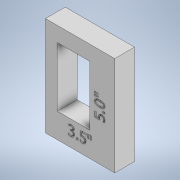
# Autodesk Inventor part: rectangular3_5x5_0-in-Template
Saved by Autodesk Inventor 2020.2 (Build 242310000, 310)
## iProperties
Created: 2020-01-27
Part Number: rectangular3_5x5_0-in-Template
Material: Generic
Document SubType Name: Modeling
Designer: robst
Density: 1 g/cm^3
Appearance: Default
Author: robst
Autodesk Inventor part; units mm, degrees
ref_plane "YZ Plane" through (0, 0, 0) normal (1, 0, 0) x (0, 1, 0)
ref_plane "XZ Plane" through (0, 0, 0) normal (0, 1, 0) x (-1, 0, 0)
ref_plane "XY Plane" through (0, 0, 0) normal (0, 0, 1) x (1, 0, 0)
sketch "Sketch1" plane through (0, 0, 0) normal (0, 0, 1) x (1, 0, 0)
  line L0 (-44.45, -63.5) -> (44.45, -63.5)
  line L1 (44.45, -63.5) -> (44.45, 63.5)
  line L2 (44.45, 63.5) -> (-44.45, 63.5)
  line L3 (-44.45, 63.5) -> (-44.45, -63.5)
  line L4 (-44.45, -63.5) -> (44.45, 63.5) construction
  line L5 (44.45, -63.5) -> (-44.45, 63.5) construction
  point P0 (0, 0)
  dimension "d0" = 88.9
  dimension "d1" = 127
  constraints: 12 end point, 2 midpoint, 2 parallel, 1 horizontal, 1 perpendicular
  measures "d0" distance of L0.start L0.end
  measures "d1" distance of L1.end L0.end
extrude "Extrusion1" add sketch "Sketch1" along normal mid plane 25.4
sketch "Sketch2" plane through (0, 0, 12.7) normal (0, 0, 1) x (1, 0, 0)
  line L0 (-44.45, 63.5) -> (-44.45, -63.5) construction
  line L1 (-44.45, -44.45) -> (44.45, -44.45) construction
  line L2 (44.45, -63.5) -> (44.45, 63.5) construction
  line L3 (-44.45, -63.5) -> (44.45, -63.5) construction
  line L4 (25.4, -63.5) -> (25.4, 63.5) construction
  spline S0 degree 2 poles (27.7156, -7.055) (28.6316, -7.055) (30.1959, -7.6416) (30.7723, -8.1768) knots 0 0 0 1 2 2 2
  spline S1 degree 2 poles (30.7723, -8.1768) (31.3486, -8.712) (32.0176, -10.3072) (32.0176, -11.2952) knots 0 0 0 1 2 2 2
  spline S2 degree 2 poles (32.0176, -11.2952) (32.0176, -12.2008) (31.6162, -13.971) (31.2972, -14.6194) knots 0 0 0 1 2 2 2
  line L5 (31.2972, -14.6194) -> (29.4961, -14.6194)
  line L6 (29.4961, -14.6194) -> (29.4961, -14.4959)
  spline S3 degree 2 poles (29.4961, -14.4959) (29.6402, -14.3004) (30.0107, -13.5697) (30.1754, -13.1271) knots 0 0 0 1 2 2 2
  spline S4 degree 2 poles (30.1754, -13.1271) (30.3503, -12.6228) (30.5459, -11.7892) (30.5459, -11.2643) knots 0 0 0 1 2 2 2
  spline S5 degree 2 poles (30.5459, -11.2643) (30.5459, -10.7497) (30.1754, -9.7823) (29.774, -9.4324) knots 0 0 0 1 2 2 2
  spline S6 degree 2 poles (29.774, -9.4324) (29.3932, -9.1133) (28.3846, -8.784) (27.7053, -8.784) knots 0 0 0 1 2 2 2
  spline S7 degree 2 poles (27.7053, -8.784) (27.0261, -8.784) (26.1616, -9.1545) (25.8734, -9.5044) knots 0 0 0 1 2 2 2
  spline S8 degree 2 poles (25.8734, -9.5044) (25.5544, -9.8646) (25.2868, -10.935) (25.2868, -11.5833) knots 0 0 0 1 2 2 2
  spline S9 degree 2 poles (25.2868, -11.5833) (25.2868, -12.2832) (25.5029, -13.6726) (25.5955, -14.0945) knots 0 0 0 1 2 2 2
  line L7 (25.5955, -14.0945) -> (19.05, -14.0945)
  line L8 (19.05, -14.0945) -> (19.05, -7.127)
  line L9 (19.05, -7.127) -> (20.5423, -7.127)
  line L10 (20.5423, -7.127) -> (20.5423, -12.4581)
  line L11 (20.5423, -12.4581) -> (23.9283, -12.4581)
  spline S10 degree 2 poles (23.9283, -12.4581) (23.8871, -12.1494) (23.8562, -11.5525) (23.8562, -11.3055) knots 0 0 0 1 2 2 2
  spline S11 degree 2 poles (23.8562, -11.3055) (23.8562, -10.3278) (24.1753, -8.9795) (24.6487, -8.362) knots 0 0 0 1 2 2 2
  spline S12 degree 2 poles (24.6487, -8.362) (25.1221, -7.7342) (26.563, -7.055) (27.7156, -7.055) knots 0 0 0 1 2 2 2
  line L12 (31.75, -2.4957) -> (31.75, -4.5335)
  line L13 (31.75, -4.5335) -> (29.3212, -4.5335)
  line L14 (29.3212, -4.5335) -> (29.3212, -2.4957)
  line L15 (29.3212, -2.4957) -> (31.75, -2.4957)
  spline S13 degree 2 poles (25.4, 7.9709) (28.8169, 7.9709) (32.0176, 5.9846) (32.0176, 3.916) knots 0 0 0 1 2 2 2
  spline S14 degree 2 poles (32.0176, 3.916) (32.0176, 1.8165) (28.7551, -0.1492) (25.4103, -0.1492) knots 0 0 0 1 2 2 2
  spline S15 degree 2 poles (25.4103, -0.1492) (21.9729, -0.1492) (18.7927, 1.8371) (18.7927, 3.916) knots 0 0 0 1 2 2 2
  spline S16 degree 2 poles (18.7927, 3.916) (18.7927, 6.0052) (22.0861, 7.9709) (25.4, 7.9709) knots 0 0 0 1 2 2 2
  spline S17 degree 2 poles (29.2697, 5.7891) (28.6419, 6.0361) (26.7071, 6.2419) (25.4, 6.2419) knots 0 0 0 1 2 2 2
  spline S18 degree 2 poles (25.4, 6.2419) (24.0929, 6.2419) (22.1684, 6.0361) (21.52, 5.7788) knots 0 0 0 1 2 2 2
  spline S19 degree 2 poles (21.52, 5.7788) (20.8716, 5.5215) (20.2027, 4.6261) (20.2027, 3.916) knots 0 0 0 1 2 2 2
  spline S20 degree 2 poles (20.2027, 3.916) (20.2027, 3.2059) (20.8716, 2.2899) (21.5406, 2.0223) knots 0 0 0 1 2 2 2
  spline S21 degree 2 poles (21.5406, 2.0223) (22.189, 1.765) (24.165, 1.5798) (25.4103, 1.5798) knots 0 0 0 1 2 2 2
  spline S22 degree 2 poles (25.4103, 1.5798) (26.7482, 1.5798) (28.539, 1.7444) (29.2388, 2.012) knots 0 0 0 1 2 2 2
  spline S23 degree 2 poles (29.2388, 2.012) (29.8975, 2.259) (30.6076, 3.175) (30.6076, 3.916) knots 0 0 0 1 2 2 2
  spline S24 degree 2 poles (30.6076, 3.916) (30.6076, 4.6158) (29.9387, 5.5318) (29.2697, 5.7891) knots 0 0 0 1 2 2 2
  line L16 (18.484, 11.501) -> (23.424, 11.1305)
  line L17 (23.424, 11.1305) -> (23.424, 10.0087)
  line L18 (23.424, 10.0087) -> (18.484, 9.6382)
  line L19 (18.484, 9.6382) -> (18.484, 11.501)
  line L20 (18.484, 14.712) -> (23.424, 14.3415)
  line L21 (23.424, 14.3415) -> (23.424, 13.2197)
  line L22 (23.424, 13.2197) -> (18.484, 12.8492)
  line L23 (18.484, 12.8492) -> (18.484, 14.712)
  spline S25 degree 2 poles (-11.3261, -39.3041) (-11.7892, -39.3041) (-12.7051, -39.5306) (-13.1477, -39.7055) knots 0 0 0 1 2 2 2
  spline S26 degree 2 poles (-13.1477, -39.7055) (-13.5594, -39.8805) (-14.1666, -40.251) (-14.4033, -40.4156) knots 0 0 0 1 2 2 2
  line L24 (-14.4033, -40.4156) -> (-14.5062, -40.4156)
  line L25 (-14.5062, -40.4156) -> (-14.5062, -38.6146)
  spline S27 degree 2 poles (-14.5062, -38.6146) (-13.9504, -38.3161) (-12.0465, -37.8324) (-11.1923, -37.8324) knots 0 0 0 1 2 2 2
  spline S28 degree 2 poles (-11.1923, -37.8324) (-10.3278, -37.8324) (-9.0413, -38.1823) (-8.5164, -38.5528) knots 0 0 0 1 2 2 2
  spline S29 degree 2 poles (-8.5164, -38.5528) (-7.9607, -38.9542) (-7.3843, -40.1172) (-7.3843, -40.8994) knots 0 0 0 1 2 2 2
  spline S30 degree 2 poles (-7.3843, -40.8994) (-7.3843, -41.9491) (-8.7634, -43.534) (-9.7308, -43.7399) knots 0 0 0 1 2 2 2
  line L26 (-9.7308, -43.7399) -> (-9.7308, -43.8634)
  spline S31 degree 2 poles (-9.7308, -43.8634) (-9.3295, -43.9457) (-8.4135, -44.3162) (-8.0224, -44.6867) knots 0 0 0 1 2 2 2
  spline S32 degree 2 poles (-8.0224, -44.6867) (-7.6313, -45.0469) (-7.1373, -46.1996) (-7.1373, -47.0332) knots 0 0 0 1 2 2 2
  spline S33 degree 2 poles (-7.1373, -47.0332) (-7.1373, -47.8874) (-7.7239, -49.3386) (-8.2591, -49.8943) knots 0 0 0 1 2 2 2
  spline S34 degree 2 poles (-8.2591, -49.8943) (-8.8149, -50.4707) (-10.3895, -51.0676) (-11.3878, -51.0676) knots 0 0 0 1 2 2 2
  spline S35 degree 2 poles (-11.3878, -51.0676) (-12.3449, -51.0676) (-14.218, -50.6045) (-14.8561, -50.2854) knots 0 0 0 1 2 2 2
  line L27 (-14.8561, -50.2854) -> (-14.8561, -48.4844)
  line L28 (-14.8561, -48.4844) -> (-14.7326, -48.4844)
  spline S36 degree 2 poles (-14.7326, -48.4844) (-14.1974, -48.8754) (-12.3861, -49.5959) (-11.4907, -49.5959) knots 0 0 0 1 2 2 2
  spline S37 degree 2 poles (-11.4907, -49.5959) (-10.9658, -49.5959) (-9.9161, -49.2665) (-9.5662, -48.8857) knots 0 0 0 1 2 2 2
  spline S38 degree 2 poles (-9.5662, -48.8857) (-9.2265, -48.5049) (-8.8663, -47.5993) (-8.8663, -46.9097) knots 0 0 0 1 2 2 2
  spline S39 degree 2 poles (-8.8663, -46.9097) (-8.8663, -46.2202) (-9.2677, -45.3248) (-9.6279, -45.0675) knots 0 0 0 1 2 2 2
  spline S40 degree 2 poles (-9.6279, -45.0675) (-9.9881, -44.8102) (-10.9658, -44.6147) (-11.5422, -44.6147) knots 0 0 0 1 2 2 2
  line L29 (-11.5422, -44.6147) -> (-12.2626, -44.6147)
  line L30 (-12.2626, -44.6147) -> (-12.2626, -43.2047)
  line L31 (-12.2626, -43.2047) -> (-11.6966, -43.2047)
  spline S41 degree 2 poles (-11.6966, -43.2047) (-10.5542, -43.2047) (-9.1133, -42.1138) (-9.1133, -41.0743) knots 0 0 0 1 2 2 2
  spline S42 degree 2 poles (-9.1133, -41.0743) (-9.1133, -40.5906) (-9.4838, -39.9011) (-9.7823, -39.6952) knots 0 0 0 1 2 2 2
  spline S43 degree 2 poles (-9.7823, -39.6952) (-10.1013, -39.4791) (-10.8835, -39.3041) (-11.3261, -39.3041) knots 0 0 0 1 2 2 2
  line L32 (-2.4957, -50.8) -> (-4.5335, -50.8)
  line L33 (-4.5335, -50.8) -> (-4.5335, -48.3712)
  line L34 (-4.5335, -48.3712) -> (-2.4957, -48.3712)
  line L35 (-2.4957, -48.3712) -> (-2.4957, -50.8)
  spline S44 degree 2 poles (7.7651, -46.7656) (7.7651, -47.6816) (7.1785, -49.2459) (6.6433, -49.8223) knots 0 0 0 1 2 2 2
  spline S45 degree 2 poles (6.6433, -49.8223) (6.1081, -50.3986) (4.5129, -51.0676) (3.5249, -51.0676) knots 0 0 0 1 2 2 2
  spline S46 degree 2 poles (3.5249, -51.0676) (2.6192, -51.0676) (0.8491, -50.6662) (0.2007, -50.3472) knots 0 0 0 1 2 2 2
  line L36 (0.2007, -50.3472) -> (0.2007, -48.5461)
  line L37 (0.2007, -48.5461) -> (0.3242, -48.5461)
  spline S47 degree 2 poles (0.3242, -48.5461) (0.5197, -48.6902) (1.2504, -49.0607) (1.693, -49.2254) knots 0 0 0 1 2 2 2
  spline S48 degree 2 poles (1.693, -49.2254) (2.1973, -49.4003) (3.0309, -49.5959) (3.5558, -49.5959) knots 0 0 0 1 2 2 2
  spline S49 degree 2 poles (3.5558, -49.5959) (4.0704, -49.5959) (5.0378, -49.2254) (5.3877, -48.824) knots 0 0 0 1 2 2 2
  spline S50 degree 2 poles (5.3877, -48.824) (5.7068, -48.4432) (6.0361, -47.4346) (6.0361, -46.7553) knots 0 0 0 1 2 2 2
  spline S51 degree 2 poles (6.0361, -46.7553) (6.0361, -46.0761) (5.6656, -45.2116) (5.3157, -44.9234) knots 0 0 0 1 2 2 2
  spline S52 degree 2 poles (5.3157, -44.9234) (4.9555, -44.6044) (3.8851, -44.3368) (3.2368, -44.3368) knots 0 0 0 1 2 2 2
  spline S53 degree 2 poles (3.2368, -44.3368) (2.5369, -44.3368) (1.1475, -44.5529) (0.7256, -44.6455) knots 0 0 0 1 2 2 2
  line L38 (0.7256, -44.6455) -> (0.7256, -38.1)
  line L39 (0.7256, -38.1) -> (7.6931, -38.1)
  line L40 (7.6931, -38.1) -> (7.6931, -39.5923)
  line L41 (7.6931, -39.5923) -> (2.362, -39.5923)
  line L42 (2.362, -39.5923) -> (2.362, -42.9783)
  spline S54 degree 2 poles (2.362, -42.9783) (2.6707, -42.9371) (3.2676, -42.9062) (3.5146, -42.9062) knots 0 0 0 1 2 2 2
  spline S55 degree 2 poles (3.5146, -42.9062) (4.4923, -42.9062) (5.8406, -43.2253) (6.4581, -43.6987) knots 0 0 0 1 2 2 2
  spline S56 degree 2 poles (6.4581, -43.6987) (7.0859, -44.1721) (7.7651, -45.613) (7.7651, -46.7656) knots 0 0 0 1 2 2 2
  line L43 (11.501, -37.534) -> (11.1305, -42.474)
  line L44 (11.1305, -42.474) -> (10.0087, -42.474)
  line L45 (10.0087, -42.474) -> (9.6382, -37.534)
  line L46 (9.6382, -37.534) -> (11.501, -37.534)
  line L47 (14.712, -37.534) -> (14.3415, -42.474)
  line L48 (14.3415, -42.474) -> (13.2197, -42.474)
  line L49 (13.2197, -42.474) -> (12.8492, -37.534)
  line L50 (12.8492, -37.534) -> (14.712, -37.534)
  point P0 (0, 0)
  dimension "d4" = 19.05
  dimension "d5" = 19.05
  constraints: 4 end point, 3 point on line, 2 horizontal, 2 vertical
  measures "d4" distance between parallel lines of L1 L3
  measures "d5" distance between parallel lines of L4 L2
extrude "Extrusion2" cut sketch "Sketch2" against normal blind 2.54
sketch "Sketch3" plane through (0, 0, 12.7) normal (0, 0, 1) x (1, 0, 0)
  line L0 (-29.21, -31.75) -> (12.7, -31.75)
  line L1 (12.7, -31.75) -> (12.7, 44.45)
  line L2 (12.7, 44.45) -> (-29.21, 44.45)
  line L3 (-29.21, 44.45) -> (-29.21, -31.75)
  line L4 (-44.45, 63.5) -> (-44.45, -63.5) projected
  line L5 (44.45, 63.5) -> (-44.45, 63.5) projected
  line L6 (44.45, -63.5) -> (44.45, 63.5) projected
  line L7 (-44.45, -63.5) -> (44.45, -63.5) projected
  point P0 (0, 0)
  dimension "d8" = 19.05
  dimension "d9" = 31.75
  dimension "d10" = 15.24
  dimension "d11" = 31.75
  constraints: 8 end point, 6 parallel, 1 horizontal, 1 perpendicular
  measures "d8" distance between parallel lines of L2 L5
  measures "d9" distance between parallel lines of L7 L0
  measures "d10" distance between parallel lines of L3 L4
  measures "d11" distance between parallel lines of L6 L1
extrude "Extrusion3" cut sketch "Sketch3" against normal through all contours L3 L2 L1 L0
body "Solid1"
